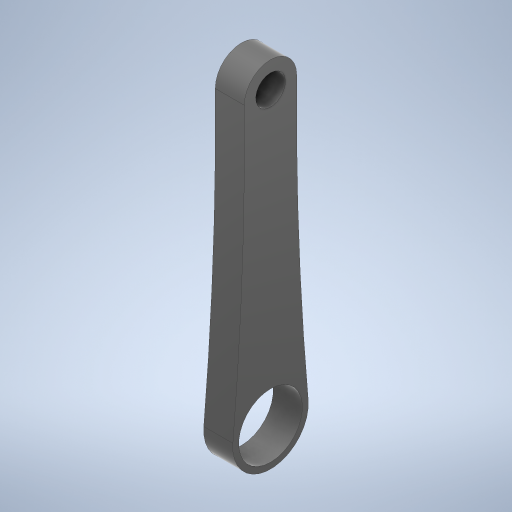
# Autodesk Inventor part: Hebel
Saved by Autodesk Inventor 2023 (Build 270158000, 158)
## iProperties
Created: 2024-01-25
Part Number: Hebel
Material: Generisch
Document SubType Name: Modeling
Designer: phili
Density: 1 g/cm^3
Appearance: Vorgabe
Author: phili
Autodesk Inventor part; units mm, degrees
ref_plane "YZ Plane" through (0, 0, 0) normal (1, 0, 0) x (0, 1, 0)
ref_plane "XZ Plane" through (0, 0, 0) normal (0, 1, 0) x (-1, 0, 0)
sketch "Skizze1" plane through (0, 0, 0) normal (1, 0, 0) x (0, 1, 0)
  circle A0 centre (-99.913, 0) radius 13
  circle A1 centre (-99.913, 0) radius 10.95
  circle A2 centre (0, 0) radius 9
  arc A3 (-98.7442, 12.9473) -> (-0.0904, 8.9995) centre (-10, 995.9932) ccw
  arc A4 (-0.0904, -8.9995) -> (-98.7442, -12.9473) centre (-10, -995.9932) ccw
  circle A5 centre (0, 0) radius 5.1
  dimension "d0" = 26
  dimension "d1" = 99.913
  dimension "d2" = 21.9
  dimension "d3" = 18
  dimension "d6" = 0
  dimension "d7" = 0
  dimension "d8" = 0
  dimension "d9" = 10
  dimension "d10" = 10
  dimension "d11" = 10.2
  constraints: 8 point on circle, 6 centre point, 4 tangent, 2 coincident
  measures "d0" diameter of A0
  measures "d1" distance of A0.centre point (0, 0)
  measures "d2" diameter of A1
  measures "d3" diameter of A2
  measures "d6" distance of A2.centre point (0, 0)
  measures "d7" vertical distance of point (0, 0) A1.centre
  measures "d8" distance of point (0, 0) A2.centre
  measures "d9" horizontal distance of point (0, 0) A3.centre
  measures "d10" horizontal distance of point (0, 0) A4.centre
  measures "d11" diameter of A5
extrude "Extrusion1" add sketch "Skizze1" along normal blind 10
ref_plane "Arbeitsebene1" through (0, 0, 0) normal (0, 0, 1) x (1, 0, 0)
